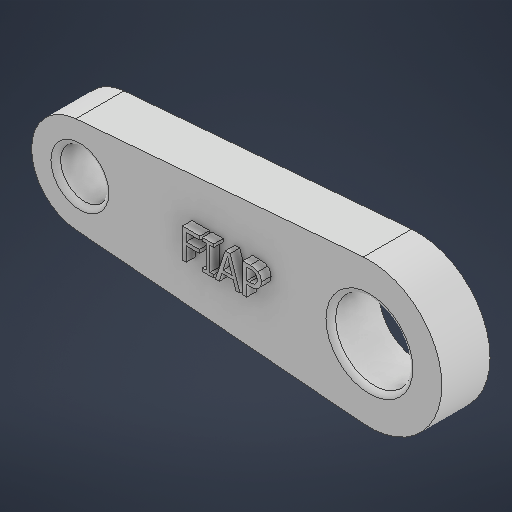
# Autodesk Inventor part: braço do robo
Saved by Autodesk Inventor 2026.2 (Build 302298010, 298A)
## iProperties
Created: 2026-08-27
Part Number: braço do robo
Material: Genérico
Document SubType Name: Modeling
Designer: Matheus
Density: 1 g/cm^3
Appearance: Padrão
Author: Matheus
Autodesk Inventor part; units mm, degrees
ref_plane "YZ Plane" through (0, 0, 0) normal (1, 0, 0) x (0, 1, 0)
ref_plane "XZ Plane" through (0, 0, 0) normal (0, 1, 0) x (-1, 0, 0)
ref_plane "XY Plane" through (0, 0, 0) normal (0, 0, 1) x (1, 0, 0)
sketch "Esboço1" plane through (0, 0, 0) normal (0, 0, 1) x (1, 0, 0)
  arc A0 (-0.4167, 4.9826) -> (-0.4167, -4.9826) centre (0, 0) ccw
  line L0 (0, 0) -> (30, 0) construction
  arc A1 (29.375, -7.4739) -> (29.375, 7.4739) centre (30, 0) ccw
  line L1 (-0.4167, 4.9826) -> (29.375, 7.4739)
  line L2 (-0.4167, -4.9826) -> (29.375, -7.4739)
  circle A2 centre (0, 0) radius 2.5
  circle A3 centre (30, 0) radius 4
  line L3 (12.0692, 0.0325) -> (20.6451, 0.0325) construction
  line L4 (20.6451, 0.0325) -> (20.6451, -3.0155) construction
  line L5 (20.6451, -3.0155) -> (12.0692, -3.0155) construction
  line L6 (12.0692, -3.0155) -> (12.0692, 0.0325) construction
  dimension "d0" = 10
  dimension "d1" = 15
  dimension "d2" = 30
  dimension "d3" = 5
  dimension "d4" = 8
  constraints: 6 end point, 4 centre point, 4 coincident, 4 point on circle, 4 tangent, 1 horizontal, 2 other
  measures "d0" diameter of A0
  measures "d1" diameter of A1
  measures "d2" distance of L0.start L0.end
  measures "d3" diameter of A2
  measures "d4" diameter of A3
extrude "Extrusão1" add sketch "Esboço1" along normal mid plane 5
sketch "Esboço2" plane through (0, 0, 2.5) normal (0, 0, 1) x (1, 0, 0)
  line L0 (11.3094, 1.8749) -> (18.1669, 1.8749) construction
  line L1 (18.1669, 1.8749) -> (18.1669, 2.829) construction
  line L2 (18.1669, 2.829) -> (11.3094, 2.829) construction
  line L3 (11.3094, 2.829) -> (11.3094, 1.8749) construction
  circle A0 centre (30, 0) radius 4 projected
  line L4 (13.441, 1.5143) -> (12.0232, 1.5143)
  line L5 (12.0232, 1.5143) -> (12.0232, 0.6547)
  line L6 (12.0232, 0.6547) -> (13.3818, 0.6547)
  line L7 (13.3818, 0.6547) -> (13.3818, 0.2941)
  line L8 (13.3818, 0.2941) -> (12.0232, 0.2941)
  line L9 (12.0232, 0.2941) -> (12.0232, -1.1731)
  line L10 (12.0232, -1.1731) -> (11.6182, -1.1731)
  line L11 (11.6182, -1.1731) -> (11.6182, 1.8749)
  line L12 (11.6182, 1.8749) -> (13.441, 1.8749)
  line L13 (13.441, 1.8749) -> (13.441, 1.5143)
  line L14 (14.8662, -1.1731) -> (13.6856, -1.1731)
  line L15 (13.6856, -1.1731) -> (13.6856, -0.8619)
  line L16 (13.6856, -0.8619) -> (14.0734, -0.8619)
  line L17 (14.0734, -0.8619) -> (14.0734, 1.5637)
  line L18 (14.0734, 1.5637) -> (13.6856, 1.5637)
  line L19 (13.6856, 1.5637) -> (13.6856, 1.8749)
  line L20 (13.6856, 1.8749) -> (14.8662, 1.8749)
  line L21 (14.8662, 1.8749) -> (14.8662, 1.5637)
  line L22 (14.8662, 1.5637) -> (14.4784, 1.5637)
  line L23 (14.4784, 1.5637) -> (14.4784, -0.8619)
  line L24 (14.4784, -0.8619) -> (14.8662, -0.8619)
  line L25 (14.8662, -0.8619) -> (14.8662, -1.1731)
  line L26 (15.0391, -1.1731) -> (16.0667, 1.8749)
  line L27 (16.0667, 1.8749) -> (16.5656, 1.8749)
  line L28 (16.5656, 1.8749) -> (17.5931, -1.1731)
  line L29 (17.5931, -1.1731) -> (17.1658, -1.1731)
  line L30 (17.1658, -1.1731) -> (16.8892, -0.3209)
  line L31 (16.8892, -0.3209) -> (15.7258, -0.3209)
  line L32 (15.7258, -0.3209) -> (15.4492, -1.1731)
  line L33 (15.4492, -1.1731) -> (15.0391, -1.1731)
  line L34 (16.778, 0.0249) -> (16.3063, 1.46)
  line L35 (16.3063, 1.46) -> (15.837, 0.0249)
  line L36 (15.837, 0.0249) -> (16.778, 0.0249)
  spline S0 degree 2 poles (19.8087, 0.9561) (19.8087, 0.7585) (19.6679, 0.4028) (19.542, 0.2793) knots 0 0 0 1 2 2 2
  spline S1 degree 2 poles (19.542, 0.2793) (19.3839, 0.1237) (18.9566, -0.0369) (18.6305, -0.0369) knots 0 0 0 1 2 2 2
  line L37 (18.6305, -0.0369) -> (18.2872, -0.0369)
  line L38 (18.2872, -0.0369) -> (18.2872, -1.1731)
  line L39 (18.2872, -1.1731) -> (17.8821, -1.1731)
  line L40 (17.8821, -1.1731) -> (17.8821, 1.8749)
  line L41 (17.8821, 1.8749) -> (18.6478, 1.8749)
  spline S2 degree 2 poles (18.6478, 1.8749) (18.9195, 1.8749) (19.2999, 1.786) (19.4456, 1.6847) knots 0 0 0 1 2 2 2
  spline S3 degree 2 poles (19.4456, 1.6847) (19.6161, 1.5686) (19.8087, 1.2105) (19.8087, 0.9561) knots 0 0 0 1 2 2 2
  spline S4 degree 2 poles (19.3864, 0.9437) (19.3864, 1.1018) (19.2777, 1.334) (19.1665, 1.4081) knots 0 0 0 1 2 2 2
  spline S5 degree 2 poles (19.1665, 1.4081) (19.0702, 1.4723) (18.8133, 1.5242) (18.6231, 1.5242) knots 0 0 0 1 2 2 2
  line L42 (18.6231, 1.5242) -> (18.2872, 1.5242)
  line L43 (18.2872, 1.5242) -> (18.2872, 0.3089)
  line L44 (18.2872, 0.3089) -> (18.5639, 0.3089)
  spline S6 degree 2 poles (18.5639, 0.3089) (18.8109, 0.3089) (19.1147, 0.388) (19.2135, 0.4917) knots 0 0 0 1 2 2 2
  spline S7 degree 2 poles (19.2135, 0.4917) (19.3049, 0.5831) (19.3864, 0.798) (19.3864, 0.9437) knots 0 0 0 1 2 2 2
  point P0 (0, 0)
  dimension "d2" = 30
  constraints: 2 other
emboss "Relevo1" sketch "Esboço2" operation add depth 1 direction (0, 0, -1) contours L4 L5 L6 L7 L8 L9 L10 L11 L12 L13 | L14 L15 L16 L17 L18 L19 L20 L21 L22 L23 L24 L25 | L26 L27 L28 L29 L30 L31 L32 L33 | S0 S1 L37 L38 L39 L40 L41 S2 S3
fillet "Arredondamento1" radius 0.5 1 edges at (-2.5, 0, 2.5)
fillet "Arredondamento2" radius 0.5 1 edges at (26, 0, 2.5)
